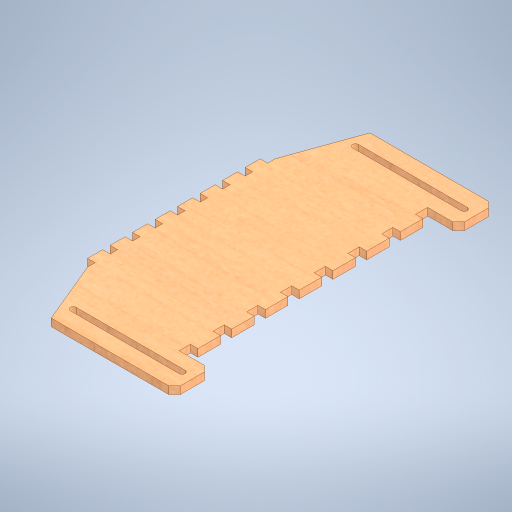
# Autodesk Inventor part: ребро_электроника
Saved by Autodesk Inventor 2023.1 (Build 271208000, 208)
## iProperties
Created: 2026-02-21
Part Number: ребро_электроника
Material: Типовые
Document SubType Name: Modeling
Designer: DELL
Density: 1 g/cm^3
Appearance: Вишневое дерево — натуральный — со слабым глянцем
Author: DELL
Autodesk Inventor part; units mm, degrees
ref_plane "YZ Plane" through (0, 0, 0) normal (1, 0, 0) x (0, 1, 0)
ref_plane "XZ Plane" through (0, 0, 0) normal (0, 1, 0) x (-1, 0, 0)
ref_plane "XY Plane" through (0, 0, 0) normal (0, 0, 1) x (1, 0, 0)
sketch "Эскиз1" plane through (0, 0, 0) normal (0, 1, 0) x (-1, 0, 0)
  line L0 (-37.5, 85.25) -> (37.5, 85.25)
  line L1 (37.5, 85.25) -> (37.5, -85.25)
  line L2 (37.5, -85.25) -> (-37.5, -85.25)
  line L3 (-37.5, -85.25) -> (-37.5, 85.25)
  line L4 (-37.5, 85.25) -> (37.5, -85.25) construction
  line L5 (37.5, 85.25) -> (-37.5, -85.25) construction
  circle A0 centre (21.5, 75.25) radius 1.6 construction
  circle A1 centre (-26.5, 75.25) radius 1.6 construction
  line L6 (37.5, 0) -> (0, 0) construction
  line L7 (-37.5, -85.25) -> (37.5, 85.25) construction
  circle A2 centre (21.5, -75.25) radius 1.6 construction
  circle A3 centre (-26.5, -75.25) radius 1.6 construction
  line L8 (37.5, 75.25) -> (-37.5, 75.25) construction
  line L9 (28.1, 75.25) -> (-33.1, 75.25) construction
  line L10 (26.5, 76.85) -> (-31.5, 76.85)
  line L11 (-31.5, 73.65) -> (26.5, 73.65)
  arc A4 (26.5, 73.65) -> (26.5, 76.85) centre (26.5, 75.25) ccw
  arc A5 (-31.5, 76.85) -> (-31.5, 73.65) centre (-31.5, 75.25) ccw
  line L12 (26.5, -76.85) -> (-31.5, -76.85)
  line L13 (-31.5, -73.65) -> (26.5, -73.65)
  arc A6 (26.5, -76.85) -> (26.5, -73.65) centre (26.5, -75.25) ccw
  arc A7 (-31.5, -73.65) -> (-31.5, -76.85) centre (-31.5, -75.25) ccw
  point P0 (-2.5, 75.25)
  point P1 (-33.1, -75.25)
  dimension "d0" = 170.5
  dimension "d1" = 75
  dimension "d2" = 3.2
  dimension "d4" = 10
  dimension "d5" = 3.2
  dimension "d7" = 10
  dimension "d29" = 48
  dimension "d30" = 3.2
  dimension "d32" = 5
  dimension "d33" = 5
  dimension "d59" = 6
  dimension "d60" = 10
  constraints: 30 end point, 11 point on circle, 9 symmetric about line, 8 centre point, 6 point on line, 4 midpoint, 4 tangent, 3 parallel, 2 horizontal, 2 perpendicular, 4 other
  measures "d0" distance of L2.end L0.start
  measures "d1" distance of L0.start L0.end
  measures "d2" diameter of A0
  measures "d4" distance from line of L0 A0.centre
  measures "d5" diameter of A1
  measures "d7" distance from line of L0 A1.centre
  measures "d29" distance of A1.centre A0.centre
  measures "d30" diameter of A5
  measures "d32" distance of A4.centre A0.centre
  measures "d33" distance of A1.centre A5.centre
  measures "d59" distance from line of L3 A5.centre
  measures "d60" distance between parallel lines of L0 L8
extrude "Выдавливание1" add sketch "Эскиз1" along normal blind 4
sketch "Эскиз2" plane through (0, 4, 0) normal (0, 1, 0) x (1, 0, 0)
  line L0 (33, 66.25) -> (33, -66.25) construction
  line L1 (-37.5, -85.25) -> (37.5, -85.25) projected
  line L2 (37.5, 85.25) -> (-37.5, 85.25) projected
  line L3 (21, -66.25) -> (25, -66.25)
  line L4 (25, -66.25) -> (25, -60.25)
  line L5 (25, -60.25) -> (21, -60.25)
  line L6 (21, -60.25) -> (21, -66.25)
  line L7 (21, -48.25) -> (25, -48.25)
  line L8 (21, -42.25) -> (21, -48.25)
  line L9 (25, -48.25) -> (25, -42.25)
  line L10 (25, -42.25) -> (21, -42.25)
  line L11 (21, -30.25) -> (25, -30.25)
  line L12 (21, -24.25) -> (21, -30.25)
  line L13 (25, -30.25) -> (25, -24.25)
  line L14 (25, -24.25) -> (21, -24.25)
  line L15 (21, -12.25) -> (25, -12.25)
  line L16 (21, -6.25) -> (21, -12.25)
  line L17 (25, -12.25) -> (25, -6.25)
  line L18 (25, -6.25) -> (21, -6.25)
  line L19 (21, 5.75) -> (25, 5.75)
  line L20 (21, 11.75) -> (21, 5.75)
  line L21 (25, 5.75) -> (25, 11.75)
  line L22 (25, 11.75) -> (21, 11.75)
  line L23 (21, 23.75) -> (25, 23.75)
  line L24 (21, 29.75) -> (21, 23.75)
  line L25 (25, 23.75) -> (25, 29.75)
  line L26 (25, 29.75) -> (21, 29.75)
  line L27 (21, 41.75) -> (25, 41.75)
  line L28 (21, 47.75) -> (21, 41.75)
  line L29 (25, 41.75) -> (25, 47.75)
  line L30 (25, 47.75) -> (21, 47.75)
  line L31 (21, 59.75) -> (25, 59.75)
  line L32 (25, 59.75) -> (25, 66.25)
  line L33 (25, 66.25) -> (21, 66.25)
  line L34 (21, 66.25) -> (21, 59.75)
  point P0 (27, -66.25)
  dimension "d14" = 19
  dimension "d16" = 4
  dimension "d17" = 6
  dimension "d20" = 18
  dimension "d34" = 4
  dimension "d35" = 6.5
  dimension "d36" = 12
  constraints: 66 end point, 4 parallel, 2 horizontal, 2 perpendicular, 1 vertical, 48 other
  measures "d14" distance from line of L1 point (27, -66.25)
  measures "d16" distance of L5.end L4.end
  measures "d17" distance of L4.end L3.end
  measures "d20" distance of L3.start L7.start
  measures "d34" distance of L33.end L32.end
  measures "d35" distance of L32.end L31.end
  measures "d36" distance from line of L30 L31.end
extrude "Выдавливание2" cut sketch "Эскиз2" against normal blind 10
sketch "Эскиз3" plane through (0, 4, 0) normal (0, 1, 0) x (1, 0, 0)
  line L0 (37.5, -85.25) -> (37.5, 85.25) projected
  line L1 (37.5, 66.25) -> (25, 66.25)
  line L2 (25, 66.25) -> (25, -66.25)
  line L3 (25, -66.25) -> (37.5, -66.25)
  line L4 (37.5, -66.25) -> (37.5, 66.25)
  line L5 (-26.5, -73.65) -> (31.5, -73.65) projected
  line L6 (31.5, 73.65) -> (-26.5, 73.65) projected
  line L7 (25, -24.25) -> (25, -30.25) projected
  point P0 (0, 0)
  point P1 (31.25, 66.25)
  point P2 (25, -27.25)
  point P3 (37.5, -66.25)
  point P4 (25, -66.25)
  point P5 (25, 66.25)
  dimension "d39" = 0
  constraints: 8 end point, 3 point on line, 2 midpoint, 2 parallel, 1 horizontal, 1 perpendicular
  measures "d39" distance from line of point (25, -27.25) L2
extrude "Выдавливание3" cut sketch "Эскиз3" against normal blind 10
chamfer "Фаска1" distance 3 angle 45 4 edges at (37.5, 2, 66.25) (37.5, 2, -66.25) (37.5, 2, -85.25) (37.5, 2, 85.25)
sketch "Эскиз5" plane through (0, 4, 0) normal (0, 1, 0) x (1, 0, 0)
  line L0 (-37.5, 85.25) -> (-37.5, -85.25) projected
  line L1 (-37.5, -85.25) -> (-46.1, -85.25)
  line L2 (-46.1, -85.25) -> (-46.1, 85.25)
  line L3 (-46.1, 85.25) -> (-37.5, 85.25)
  line L4 (-37.5, 85.25) -> (-37.5, -85.25)
  point P0 (0, 0)
  dimension "d61" = 8.6
  constraints: 8 end point, 2 parallel, 1 horizontal, 1 perpendicular
  measures "d61" distance of L2.end L3.end
extrude "Выдавливание5" add sketch "Эскиз5" against normal blind 4
sketch "Эскиз6" plane through (0, 4, 0) normal (0, 1, 0) x (1, 0, 0)
  line L0 (-46.1, -60) -> (-42.1, -60) construction
  line L1 (-42.1, 60) -> (-46.1, 60) construction
  line L2 (-46.1, 60) -> (-46.1, -60) construction
  line L3 (-46.1, -60) -> (-42.1, 60) construction
  line L4 (-42.1, -60) -> (-46.1, 60) construction
  line L5 (-46.1, 85.25) -> (-46.1, -85.25) construction
  line L6 (-42.1, -48) -> (-46.1, -48)
  line L7 (-46.1, -48) -> (-46.1, -52)
  line L8 (-46.1, -52) -> (-42.1, -52)
  line L9 (-42.1, -52) -> (-42.1, -48)
  line L10 (-42.1, -40) -> (-42.1, -36)
  line L11 (-46.1, -40) -> (-42.1, -40)
  line L12 (-46.1, -36) -> (-46.1, -40)
  line L13 (-42.1, -36) -> (-46.1, -36)
  line L14 (-42.1, -28) -> (-42.1, -24)
  line L15 (-46.1, -28) -> (-42.1, -28)
  line L16 (-46.1, -24) -> (-46.1, -28)
  line L17 (-42.1, -24) -> (-46.1, -24)
  line L18 (-42.1, -16) -> (-42.1, -12)
  line L19 (-46.1, -16) -> (-42.1, -16)
  line L20 (-46.1, -12) -> (-46.1, -16)
  line L21 (-42.1, -12) -> (-46.1, -12)
  line L22 (-42.1, -4) -> (-42.1, 0)
  line L23 (-46.1, -4) -> (-42.1, -4)
  line L24 (-46.1, 0) -> (-46.1, -4)
  line L25 (-42.1, 0) -> (-46.1, 0)
  line L26 (-42.1, 8) -> (-42.1, 12)
  line L27 (-46.1, 8) -> (-42.1, 8)
  line L28 (-46.1, 12) -> (-46.1, 8)
  line L29 (-42.1, 12) -> (-46.1, 12)
  line L30 (-42.1, 20) -> (-42.1, 24)
  line L31 (-46.1, 20) -> (-42.1, 20)
  line L32 (-46.1, 24) -> (-46.1, 20)
  line L33 (-42.1, 24) -> (-46.1, 24)
  line L34 (-42.1, 32) -> (-42.1, 36)
  line L35 (-46.1, 32) -> (-42.1, 32)
  line L36 (-46.1, 36) -> (-46.1, 32)
  line L37 (-42.1, 36) -> (-46.1, 36)
  line L38 (-42.1, 44) -> (-42.1, 48)
  line L39 (-46.1, 44) -> (-42.1, 44)
  line L40 (-46.1, 48) -> (-46.1, 44)
  line L41 (-42.1, 48) -> (-46.1, 48)
  point P0 (0, 0)
  point P1 (-44.1, 0)
  point P2 (-46.1, 0)
  dimension "d64" = 4
  dimension "d65" = 120
  dimension "d66" = 4
  dimension "d67" = 4
  dimension "d68" = 8
  dimension "d71" = 12
  constraints: 82 end point, 4 midpoint, 3 parallel, 2 horizontal, 1 perpendicular, 1 vertical, 64 other
  measures "d64" distance of L1.end L1.start
  measures "d65" distance of L1.start L0.end
  measures "d66" distance of L8.end L7.end
  measures "d67" distance of L7.end L6.end
  measures "d68" distance between parallel lines of L0 L8
  measures "d71" distance of L8.end L10.start
extrude "Выдавливание6" cut sketch "Эскиз6" against normal blind 4
sketch "Эскиз7" plane through (0, 4, 0) normal (0, 1, 0) x (1, 0, 0)
  line L0 (-42.1, -52) -> (-42.1, -48) projected
  line L1 (-42.1, -52) -> (-28.2738, -85.25)
  line L2 (34.5, -85.25) -> (-46.1, -85.25) projected
  line L3 (-46.1, -52) -> (-46.1, -85.25) projected
  line L4 (-46.1, -85.25) -> (-28.2738, -85.25)
  line L5 (-46.1, -85.25) -> (-46.1, -52)
  line L6 (-46.1, -52) -> (-42.1, -52)
  arc A0 (-26.5, -73.65) -> (-26.5, -76.85) centre (-26.5, -75.25) ccw projected
  line L7 (0, 0) -> (-4.0175, 0)
  line L8 (-42.1, 48) -> (-42.1, 44) projected
  line L9 (-42.1, 48) -> (-28.7698, 85.25)
  line L10 (34.5, 85.25) -> (-46.1, 85.25) projected
  line L11 (-46.1, 85.25) -> (-28.7698, 85.25)
  line L12 (-46.1, 85.25) -> (-46.1, 48)
  line L13 (-46.1, 48) -> (-42.1, 48)
  arc A1 (-26.5, 76.85) -> (-26.5, 73.65) centre (-26.5, 75.25) ccw projected
  point P0 (-28.1, -75.25)
  point P1 (-28.1, 75.25)
  dimension "d78" = 4
  dimension "d81" = 4
  constraints: 18 end point, 2 horizontal, 2 perpendicular, 2 point on circle, 2 point on line, 2 vertical, 1 collinear
  measures "d78" distance from line of L1 point (-28.1, -75.25)
  measures "d81" distance from line of L9 point (-28.1, 75.25)
extrude "Выдавливание7" cut sketch "Эскиз7" against normal blind 4
